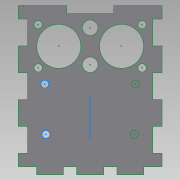
# Autodesk Inventor part: srf diag kiri
Saved by Autodesk Inventor 2015 SP1 (Build 190203100, 203)
## iProperties
Created: 2015-02-15
Part Number: srf diag kiri
Material: Generic
Document SubType Name: Modeling
Designer: Rafi Kurnia Putra
Density: 1 g/cm^3
Appearance: Default
Author: Rafi Kurnia Putra
Autodesk Inventor part; units mm, degrees
ref_plane "YZ Plane" through (0, 0, 0) normal (1, 0, 0) x (0, 1, 0)
ref_plane "XZ Plane" through (0, 0, 0) normal (0, 1, 0) x (-1, 0, 0)
ref_plane "XY Plane" through (0, 0, 0) normal (0, 0, 1) x (1, 0, 0)
sketch "Sketch1" plane through (0, 0, 0) normal (0, 0, 1) x (1, 0, 0)
  line L0 (-16.2709, 3) -> (-16.2709, 0)
  line L1 (-33.7709, 3) -> (-16.2709, 3)
  line L2 (-33.7709, 0) -> (-33.7709, 3)
  line L3 (-33.7709, 0) -> (-48.7992, 0)
  line L4 (-30.0209, 63) -> (-20.0209, 63)
  line L5 (-20.0209, 63) -> (-20.0209, 60)
  line L6 (-30.0209, 60) -> (-30.0209, 63)
  line L7 (-30.0209, 63) -> (-20.0209, 60) construction
  line L8 (-20.0209, 63) -> (-30.0209, 60) construction
  line L9 (-25.4776, 30) -> (-35.4566, 30) construction
  line L10 (-25.0209, 30) -> (-25.0209, 38) construction
  line L11 (-45.0209, 63) -> (-35.0209, 63)
  line L12 (-35.0209, 63) -> (-35.0209, 60)
  line L13 (-45.0209, 60) -> (-45.0209, 63)
  line L14 (-45.0209, 63) -> (-35.0209, 60) construction
  line L15 (-35.0209, 63) -> (-45.0209, 60) construction
  line L16 (-15.0209, 63) -> (-5.0209, 63)
  line L17 (-5.0209, 63) -> (-5.0209, 60)
  line L18 (-15.0209, 60) -> (-15.0209, 63)
  line L19 (-15.0209, 63) -> (-5.0209, 60) construction
  line L20 (-5.0209, 63) -> (-15.0209, 60) construction
  line L21 (-30.0209, 63) -> (-20.0209, 63)
  line L22 (-20.0209, 63) -> (-20.0209, 60)
  line L23 (-30.0209, 60) -> (-30.0209, 63)
  line L24 (-30.0209, 63) -> (-20.0209, 60) construction
  line L25 (-20.0209, 63) -> (-30.0209, 60) construction
  line L26 (-48.7992, 60) -> (-45.0209, 60)
  line L27 (-35.0209, 60) -> (-30.0209, 60)
  line L28 (-20.0209, 60) -> (-15.0209, 60)
  line L29 (-48.7992, 15) -> (-51.799, 15)
  line L30 (-51.799, 15) -> (-51.799, 25)
  line L31 (-51.799, 25) -> (-48.7992, 25)
  line L32 (-48.7992, 35) -> (-51.799, 35)
  line L33 (-51.799, 35) -> (-51.799, 45)
  line L34 (-48.7992, 45) -> (-51.799, 45)
  line L35 (-48.7992, 55) -> (-51.7992, 55)
  line L36 (-48.7992, 55) -> (-45.7992, 55) construction
  line L37 (-51.7992, 55) -> (-51.7992, 60)
  line L38 (-51.7992, 60) -> (-48.7992, 60)
  line L39 (-48.7992, 55) -> (-48.7992, 45)
  line L40 (-48.7992, 35) -> (-48.7992, 25)
  line L41 (-48.7992, 15) -> (-48.7992, 5)
  line L42 (-48.7992, 5) -> (-51.7992, 5)
  line L43 (-51.7992, 5) -> (-51.7992, 0)
  line L44 (-51.7992, 0) -> (-48.7992, 0)
  line L45 (-16.2709, 0) -> (-1.2426, 0)
  line L46 (-1.2426, 60) -> (-5.0209, 60)
  line L47 (-1.2426, 15) -> (1.7572, 15)
  line L48 (1.7572, 15) -> (1.7572, 25)
  line L49 (1.7572, 25) -> (-1.2426, 25)
  line L50 (-1.2426, 35) -> (1.7572, 35)
  line L51 (1.7572, 35) -> (1.7572, 45)
  line L52 (-1.2426, 45) -> (1.7572, 45)
  line L53 (-1.2426, 55) -> (1.7574, 55)
  line L54 (1.7574, 55) -> (1.7574, 60)
  line L55 (1.7574, 60) -> (-1.2426, 60)
  line L56 (-1.2426, 55) -> (-1.2426, 45)
  line L57 (-1.2426, 35) -> (-1.2426, 25)
  line L58 (-1.2426, 15) -> (-1.2426, 5)
  line L59 (-1.2426, 5) -> (1.7574, 5)
  line L60 (1.7574, 5) -> (1.7574, 0)
  line L61 (1.7574, 0) -> (-1.2426, 0)
  circle A0 centre (-44.3959, 23.1933) radius 1.5875
  circle A1 centre (-44.3959, 7.0713) radius 1.5875
  circle A2 centre (-36.7209, 15.1323) radius 8.25
  circle A3 centre (-25.0211, 22.0323) radius 2.95
  circle A4 centre (-25.0211, 8.2323) radius 2.95
  circle A5 centre (-13.3209, 15.1323) radius 8.25
  circle A6 centre (-5.6459, 7.0713) radius 1.5875
  circle A7 centre (-5.6459, 23.1933) radius 1.5875
  circle A8 centre (-41.9566, 29.25) radius 1.5
  circle A9 centre (-41.5, 48) radius 1.5
  line L62 (-5.6459, 7.0713) -> (-44.3959, 23.1933) construction
  line L63 (-44.3959, 23.1933) -> (-5.6459, 23.1933) construction
  line L64 (-5.6459, 23.1933) -> (-44.3959, 7.0713) construction
  point P0 (0, 0)
  point P1 (-25.0209, 61.5)
  point P2 (-40.0209, 61.5)
  point P3 (-10.0209, 61.5)
  point P4 (-25.0209, 61.5)
  point P5 (-48.7992, 30)
  point P6 (-1.2426, 30)
  point P7 (-25.4776, 15.3162)
  point P8 (-25.4776, 15.3162)
  point P9 (-25.4776, 15.3162)
  point P10 (-25.4776, 15.3162)
  point P11 (-25.0209, 3)
  point P12 (-25.0209, 15.1323)
  dimension "d0" = 10
  dimension "d1" = 3
  dimension "d4" = 15
  dimension "d7" = 15
  dimension "d13" = 3
  dimension "d14" = 180
  dimension "d15" = 3
  dimension "d17" = 7.675
  dimension "d18" = 7.675
  dimension "d23" = 2.9998
  dimension "d30" = 11.7002
  dimension "d31" = 11.6998
  dimension "d32" = 7.675
  dimension "d33" = 7.675
  dimension "d34" = 11.6998
  dimension "d35" = 11.7002
  dimension "d45" = 8.061
  dimension "d46" = 8.061
  constraints: 130 end point, 17 symmetric about line, 12 midpoint, 10 centre point, 9 horizontal, 7 perpendicular, 6 vertical, 5 collinear, 3 horizontal alignment, 1 coincident, 1 parallel, 1 other
  measures "d0" distance of L5.end L6.start
  measures "d1" distance of L4.end L5.end
  measures "d4" distance of L5.end L12.end
  measures "d7" distance of L5.end L17.end
  measures "d13" distance of L35.start L35.end
  measures "d14" angle of L35 L36
  measures "d15" distance of L41.end L42.end
  measures "d17" horizontal distance of L62.start A5.centre
  measures "d18" horizontal distance of A2.centre L62.end
  measures "d23" distance between parallel lines of L57 L51
  measures "d30" horizontal distance of A4.centre A5.centre
  measures "d31" horizontal distance of A4.centre A2.centre
  measures "d32" horizontal distance of A5.centre L63.end
  measures "d33" horizontal distance of A2.centre L64.end
  measures "d34" horizontal distance of A2.centre A3.centre
  measures "d35" horizontal distance of A3.centre A5.centre
  measures "d45" vertical distance of A5.centre L63.end
  measures "d46" vertical distance of L62.start A5.centre
extrude "Extrusion2" add sketch "Sketch1" along normal blind 3
sketch "Sketch2" plane through (0, 0, 3) normal (0, 0, 1) x (1, 0, 0)
  line L0 (-1.2426, 5) -> (-1.2426, 15) projected
  line L1 (-1.2426, 25) -> (-1.2426, 35) projected
  line L2 (-1.2426, 45) -> (-1.2426, 55) projected
  line L3 (-48.7992, 55) -> (-48.7992, 45) projected
  line L4 (-48.7992, 35) -> (-48.7992, 25) projected
  line L5 (-48.7992, 15) -> (-48.7992, 5) projected
  line L6 (-1.2426, 5) -> (-1.7426, 5)
  line L7 (-1.7426, 5) -> (-1.7426, 15)
  line L8 (-1.7426, 15) -> (-1.2426, 15)
  line L9 (-1.2426, 25) -> (-1.7426, 25)
  line L10 (-1.7426, 25) -> (-1.7426, 35)
  line L11 (-1.7426, 35) -> (-1.2426, 35)
  line L12 (-1.2426, 45) -> (-1.7426, 45)
  line L13 (-1.7426, 45) -> (-1.7426, 55)
  line L14 (-1.7426, 55) -> (-1.2426, 55)
  line L15 (-48.7992, 5) -> (-48.2992, 5)
  line L16 (-48.2992, 5) -> (-48.2992, 15)
  line L17 (-48.2992, 15) -> (-48.7992, 15)
  line L18 (-48.7992, 25) -> (-48.2992, 25)
  line L19 (-48.2992, 25) -> (-48.2992, 35)
  line L20 (-48.2992, 35) -> (-48.7992, 35)
  line L21 (-48.7992, 45) -> (-48.2992, 45)
  line L22 (-48.7992, 45) -> (-51.799, 45) projected
  line L23 (-48.2992, 45) -> (-48.2992, 55)
  line L24 (-48.2992, 55) -> (-48.7992, 55)
  point P0 (0, 0)
  dimension "d24" = 0.5
  dimension "d25" = 0.5
  dimension "d28" = 0.5
  dimension "d29" = 0.5
  constraints: 36 end point, 8 perpendicular, 5 horizontal, 4 point on line, 1 collinear, 1 parallel, 1 vertical
  measures "d24" distance of L0.start L6.end
  measures "d25" distance of L5.end L15.end
  measures "d28" distance of L1.start L9.end
  measures "d29" distance of L4.end L18.end
extrude "Extrusion3" cut sketch "Sketch2" against normal through all
sketch "Sketch3" plane through (0, 0, 3) normal (0, 0, 1) x (1, 0, 0)
  line L0 (-48.2992, 25) -> (-51.799, 25) projected
  line L1 (-51.799, 25) -> (-51.799, 15) projected
  line L2 (-51.799, 15) -> (-48.2992, 15) projected
  line L3 (-48.2992, 15) -> (-48.2992, 5) projected
  line L4 (-48.2992, 5) -> (-51.7992, 5) projected
  line L5 (-51.7992, 5) -> (-51.7992, 0) projected
  line L6 (-51.7992, 0) -> (-33.7709, 0) projected
  line L7 (-33.7709, 0) -> (-33.7709, 3) projected
  line L8 (-33.7709, 3) -> (-16.2709, 3) projected
  line L9 (-16.2709, 3) -> (-16.2709, 0) projected
  line L10 (-16.2709, 0) -> (1.7574, 0) projected
  line L11 (1.7574, 0) -> (1.7574, 5) projected
  line L12 (1.7574, 5) -> (-1.7426, 5) projected
  line L13 (-1.7426, 5) -> (-1.7426, 15) projected
  line L14 (-1.7426, 15) -> (1.7572, 15) projected
  line L15 (1.7572, 15) -> (1.7572, 25) projected
  line L16 (1.7572, 25) -> (-1.7426, 25) projected
  line L17 (-1.7426, 25) -> (-1.7426, 35) projected
  line L18 (-1.7426, 35) -> (1.7572, 35) projected
  line L19 (1.7572, 35) -> (1.7572, 45) projected
  line L20 (1.7572, 45) -> (-1.7426, 45) projected
  line L21 (-1.7426, 45) -> (-1.7426, 55) projected
  line L22 (-1.7426, 55) -> (1.7574, 55) projected
  line L23 (1.7574, 55) -> (1.7574, 60) projected
  line L24 (1.7574, 60) -> (-5.0209, 60) projected
  line L25 (-5.0209, 60) -> (-5.0209, 63) projected
  line L26 (-5.0209, 63) -> (-15.0209, 63) projected
  line L27 (-15.0209, 63) -> (-15.0209, 60) projected
  line L28 (-15.0209, 60) -> (-20.0209, 60) projected
  line L29 (-20.0209, 60) -> (-20.0209, 63) projected
  line L30 (-20.0209, 63) -> (-30.0209, 63) projected
  line L31 (-30.0209, 63) -> (-30.0209, 60) projected
  line L32 (-30.0209, 60) -> (-35.0209, 60) projected
  line L33 (-35.0209, 60) -> (-35.0209, 63) projected
  line L34 (-35.0209, 63) -> (-45.0209, 63) projected
  line L35 (-45.0209, 63) -> (-45.0209, 60) projected
  line L36 (-45.0209, 60) -> (-51.7992, 60) projected
  line L37 (-51.7992, 60) -> (-51.7992, 55) projected
  line L38 (-51.7992, 55) -> (-48.2992, 55) projected
  line L39 (-48.2992, 55) -> (-48.2992, 45) projected
  line L40 (-48.2992, 45) -> (-51.799, 45) projected
  line L41 (-51.799, 45) -> (-51.799, 35) projected
  line L42 (-51.799, 35) -> (-48.2992, 35) projected
  line L43 (-48.2992, 35) -> (-48.2992, 25) projected
  circle A0 centre (-13.3209, 15.1323) radius 8.25 projected
  circle A1 centre (-36.7209, 15.1323) radius 8.25 projected
  circle A2 centre (-25.0211, 8.2323) radius 2.95 projected
  circle A3 centre (-25.0211, 22.0323) radius 2.95 projected
  circle A4 centre (-5.6459, 7.0713) radius 1.5875 projected
  circle A5 centre (-5.6459, 23.1933) radius 1.5875 projected
  circle A6 centre (-44.3959, 7.0713) radius 1.5875 projected
  circle A7 centre (-44.3959, 23.1933) radius 1.5875 projected
  circle A8 centre (-41.9566, 29.25) radius 1.5 projected
  circle A9 centre (-41.5, 48) radius 1.5 projected
  line L44 (-25.0211, 33) -> (-25.0211, 49.5)
  circle A10 centre (-8.0855, 29.25) radius 1.5
  circle A11 centre (-8.5422, 48) radius 1.5
  point P0 (0, 0)
  constraints: 2 centre point, 2 end point, 2 symmetric about line, 1 vertical, 2 other
extrude "Extrusion4" cut sketch "Sketch3" against normal up to next contours A10 | A11
extrude "Extrusion5" add sketch "Sketch3" against normal blind 3 contours A8 | A9
equation "\"d46\" = d45"
equation "\"d25\" = d24"
equation "\"d28\" = d24"
equation "\"d29\" = d24"
body "Solid2"
